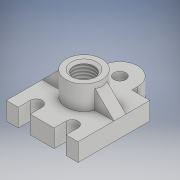
# Autodesk Inventor part: Деталь5-19
Saved by Autodesk Inventor 2019 (Build 230136000, 136)
## iProperties
Created: 2020-04-05
Part Number: Деталь5-19
Material: Типовые
Document SubType Name: Modeling
Designer: Diana
Density: 1 g/cm^3
Appearance: По умолчанию
Mass: 64.2878 g
Surface Area: 163.412 cm^2
Volume: 64.2878 cm^3
Author: Diana
Autodesk Inventor part; units mm, degrees
ref_plane "YZ Plane" through (0, 0, 0) normal (1, 0, 0) x (0, 1, 0)
ref_plane "XZ Plane" through (0, 0, 0) normal (0, 1, 0) x (-1, 0, 0)
sketch "Эскиз1" plane through (0, 0, 0) normal (0, 1, 0) x (-1, 0, 0)
  line L0 (-30, -30) -> (30, -30)
  line L1 (30, -30) -> (30, 30)
  line L2 (30, 30) -> (-30, 30)
  line L3 (-30, 30) -> (-30, -30)
  line L4 (-30, -30) -> (30, 30) construction
  line L5 (30, -30) -> (-30, 30) construction
  line L6 (20, 20) -> (20, 30)
  line L7 (10, 30) -> (10, 20)
  line L8 (10, 20) -> (20, 30) construction
  line L9 (20, 20) -> (10, 30) construction
  line L10 (0, -66) -> (0, 46) projected
  line L11 (-10, 30) -> (-20, 30)
  line L12 (-20, 30) -> (-20, 20)
  line L13 (-10, 20) -> (-10, 30)
  line L14 (-10, 30) -> (-20, 20) construction
  line L15 (-20, 30) -> (-10, 20) construction
  line L16 (42, 0) -> (-42, 0) projected
  arc A0 (-20, 20) -> (-10, 20) centre (-15, 20) ccw
  arc A1 (10, 20) -> (20, 20) centre (15, 20) ccw
  line L17 (20, 30) -> (10, 30)
  circle A2 centre (0, -35) radius 5
  line L18 (15, -35) -> (15, -30)
  line L19 (-15, -35) -> (-15, -30)
  arc A3 (-15, -35) -> (15, -35) centre (0, -35) ccw
  point P0 (0, 0)
  point P1 (15, 25)
  point P2 (-15, 25)
  dimension "d0" = 60
  dimension "d1" = 60
  dimension "d4" = 30
  dimension "d5" = 30
  dimension "d7" = 10
  dimension "d9" = 10
  dimension "d14" = 10
  dimension "d15" = 5
  dimension "d41" = 15
  dimension "d42" = 10
  dimension "d43" = 10
  dimension "d44" = 5
  constraints: 36 end point, 6 midpoint, 6 point on circle, 4 centre point, 4 parallel, 4 perpendicular, 3 point on line, 3 tangent, 2 horizontal, 1 collinear
  measures "d0" distance of L2.end L1.end
  measures "d1" distance of L0.end L1.end
  measures "d4" distance of point (-15, 25) point (15, 25)
  measures "d5" distance between parallel lines of L16 L11
  measures "d7" distance between parallel lines of L7 L6
  measures "d9" distance between parallel lines of L12 L13
  measures "d14" diameter of A2
  measures "d15" distance from line of L0 A2.centre
  measures "d41" distance from line of L10 point (15, 25)
  measures "d42" distance of L13.start L11.start
  measures "d43" distance of L11.end L12.end
  measures "d44" radius of A0
extrude "Выдавливание1" add sketch "Эскиз1" along normal blind 15 contours L3 L16 L10 L0 | L0 A2 L10 A3 L19 | L3 L2 L12 A0 L13 L10 L16 | L10 L16 L1 L0 | L0 L18 A3 L10 A2 | L10 L2 L7 A1 L6 L1 L16
sketch "Эскиз2" plane through (0, 15, 0) normal (0, 1, 0) x (1, 0, 0)
  circle A0 centre (0, 5) radius 15
  line L0 (0, 66) -> (0, -46) projected
  line L1 (30, 30) -> (-30, 30) projected
  point P0 (0, 0)
  point P1 (-14.1421, 30)
  dimension "d18" = 30
  dimension "d19" = 25
  constraints: 1 centre point, 1 point on line
  measures "d18" diameter of A0
  measures "d19" distance from line of L1 A0.centre
extrude "Выдавливание2" add sketch "Эскиз2" along normal blind 20
sketch "Эскиз3" plane through (0, 35, -5) normal (0, 1, 0) x (1, 0, 0)
  circle A0 centre (0, 0) radius 15 projected
  point P0 (0, -5)
hole "Отверстие1" at (0, 35, -5) direction (0, -1, 0) diameter 17.294 end through all thread size "M20x2.5" designation "M20" class "6H" standard "GB Metric profile"
chamfer "Фаска1" distance 2 angle 45 1 edges at (0, 35, -13.647)
sketch "Эскиз4" plane through (0, 35, -5) normal (0, 1, 0) x (1, 0, 0)
  circle A0 centre (0, 0) radius 15 projected
  point P0 (0, -5)
ref_plane "РабПлоскость1" through (0, 0, -5) normal (0, 0, 1) x (1, 0, 0)
sketch "Эскиз5" plane through (0, 0, -5) normal (0, 0, 1) x (1, 0, 0)
  line L0 (15, 15) -> (15, 35) projected
  line L1 (30, 15) -> (15, 15) projected
  line L2 (15, 30) -> (30, 15)
  point P0 (0, 0)
  point P1 (14.1421, 15)
  dimension "d33" = 5
  constraints: 2 end point, 1 point on line
  measures "d33" distance of L0.end L2.start
extrude "Ребро жесткости1" add sketch "Эскиз5" along normal mid plane 10 rib yes fills toward (22.4646, 22.4646) open curves L2
mirror "Зеркальное отражение1" about plane through (0, 0, 0) normal (1, 0, 0) of "Ребро жесткости1"
